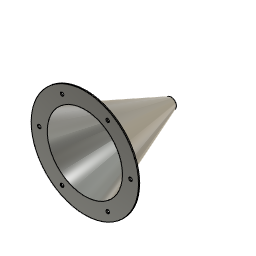
cone (Autodesk Fusion 360 design; units mm, degrees)
Autodesk Fusion 360 part; units mm, degrees
sketch "Esquisse1" plane through (0, 0, 0) normal (0, 0, 1) x (1, 0, 0)
  line L0 (0, 0) -> (0, 80)
  line L1 (0, 0) -> (50, 0) construction
  line L2 (50, 0) -> (50, 1)
  line L3 (50, 1) -> (35.685, 1)
  line L4 (35.685, 1) -> (4.9324, 80.3613)
  line L5 (4, 80) -> (35, 0)
  line L6 (35, 0) -> (50, 0)
  line L7 (4.9324, 80.3613) -> (4, 80)
  line L8 (4, 80) -> (0, 80) construction
  dimension "d1" = 1
  dimension "d2" = 35
  dimension "d3" = 15
  dimension "d4" = 4
  dimension "d5" = 80
  constraint coincident L0.start L1.start
  constraint vertical L0
  constraint perpendicular L0 L1
  constraint perpendicular L1 L2
  constraint perpendicular L2 L3
  constraint coincident L1 L5.end
  constraint parallel L4 L5
  constraint perpendicular L5 L7
  constraint horizontal L8
  constraint equal L2 L7
  measures "d1" distance of L1.end L2.end
  measures "d2" distance of L0.start L5.end
  measures "d3" distance of L1.end L5.end
  measures "d4" distance of L0.end L5.start
  measures "d5" distance of L0.start L0.end
revolve "Révolution1" add sketch "Esquisse1" angle 360 about axis through (0, 0, 0) along (0, 1, 0)
sketch "Esquisse2" plane through (0, 0, 0) normal (0, -1, 0) x (1, 0, 0)
  circle A0 centre (0, 0) radius 50
  circle A1 centre (0, 0) radius 35
  line L0 (21.25, 36.8061) -> (-21.25, 36.8061) construction
  line L1 (-21.25, 36.8061) -> (-42.5, 0) construction
  line L2 (-42.5, 0) -> (-21.25, -36.8061) construction
  line L3 (-21.25, -36.8061) -> (21.25, -36.8061) construction
  line L4 (21.25, -36.8061) -> (42.5, 0) construction
  line L5 (42.5, 0) -> (21.25, 36.8061) construction
  line L6 (-50, 0) -> (50, 0) construction
  circle A2 centre (0, 0) radius 42.5 construction
  circle A3 centre (-21.25, 36.8061) radius 1.6
  circle A4 centre (21.25, 36.8061) radius 1.6
  circle A5 centre (42.5, 0) radius 1.6
  circle A6 centre (21.25, -36.8061) radius 1.6
  circle A7 centre (-21.25, -36.8061) radius 1.6
  circle A8 centre (-42.5, 0) radius 1.6
  dimension "d7" = 7.5
  dimension "d8" = 3.2
  constraint coincident A0.centre A1.centre
  constraint coincident A0 L6.start
  constraint coincident A0 L6.end
  constraint horizontal L6
  constraint coincident L4.end L6
  constraint coincident A0.centre L6
  constraint coincident L0.end A2
  constraint coincident L0.end L1.start
  constraint coincident L0.start L5.end
  constraint coincident L4.end L5.start
  constraint coincident L3.end L4.start
  constraint coincident L2.end L3.start
  constraint coincident L1.end L2.start
  constraint equal A3 A4
  constraint equal A4 A5
  constraint equal A5 A6
  constraint equal A6 A7
  constraint equal A7 A8
  measures "d7" distance of A1 A2
  measures "d8" diameter of A3
extrude "Extrusion1" cut sketch "Esquisse2" against normal through all contours A3 | A4 | A5 | A6 | A7 | A8
equation "d2 = ( 70 / 2 ) * 1 mm"
